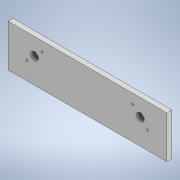
# Autodesk Inventor part: Indexer Upper Plate
Saved by Autodesk Inventor 2020 (Build 240168000, 168)
## iProperties
Created: 2020-02-02
Part Number: Indexer Upper Plate
Material: Generic
Document SubType Name: Modeling
Designer: JimAndVal
Density: 1 g/cm^3
Appearance: Default
Author: JimAndVal
Autodesk Inventor part; units mm, degrees
ref_plane "YZ Plane" through (0, 0, 0) normal (1, 0, 0) x (0, 1, 0)
ref_plane "XZ Plane" through (0, 0, 0) normal (0, 1, 0) x (-1, 0, 0)
ref_plane "XY Plane" through (0, 0, 0) normal (0, 0, 1) x (1, 0, 0)
sketch "Sketch1" plane through (0, 0, 0) normal (0, 0, 1) x (1, 0, 0)
  line L0 (-190.5, 50.8) -> (190.5, 50.8)
  line L1 (190.5, 50.8) -> (190.5, -50.8)
  line L2 (190.5, -50.8) -> (-190.5, -50.8)
  line L3 (-190.5, -50.8) -> (-190.5, 50.8)
  line L4 (-190.5, 50.8) -> (190.5, -50.8) construction
  line L5 (190.5, 50.8) -> (-190.5, -50.8) construction
  circle A0 centre (-127, 10.16) radius 9.525
  circle A1 centre (-109.0422, 28.1178) radius 2.3812
  circle A2 centre (-144.9578, -7.7978) radius 2.3812
  line L6 (0, 0) -> (0, 83.7438) construction
  circle A3 centre (127, 10.16) radius 9.525
  circle A4 centre (109.0422, 28.1178) radius 2.3812
  circle A5 centre (144.9578, -7.7978) radius 2.3812
  dimension "d0" = 381
  dimension "d1" = 101.6
  dimension "d2" = 19.05
  dimension "d4" = 127
  dimension "d5" = 60.96
  dimension "d6" = 4.7625
  dimension "d8" = 17.9578
  dimension "d9" = 17.9578
  dimension "d10" = 4.7625
  dimension "d11" = 17.9578
  dimension "d12" = 17.9578
  constraints: 14 end point, 6 centre point, 3 symmetric about line, 2 midpoint, 2 parallel, 1 horizontal, 1 perpendicular, 1 vertical, 3 other
  measures "d0" distance of L1.end L2.end
  measures "d1" distance of L0.end L1.end
  measures "d2" diameter of A0
  measures "d4" horizontal distance of A0.centre L6.start
  measures "d5" distance from line of L2 A0.centre
  measures "d6" diameter of A1
  measures "d8" horizontal distance of A0.centre A1.centre
  measures "d9" horizontal distance of A1.centre A0.centre
  measures "d10" diameter of A2
  measures "d11" horizontal distance of A2.centre A0.centre
  measures "d12" horizontal distance of A0.centre A2.centre
extrude "Extrusion1" add sketch "Sketch1" along normal mid plane 11.999
body "Solid1"
